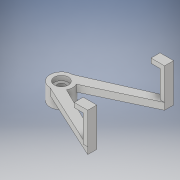
# Autodesk Inventor part: microphone_fix
Saved by Autodesk Inventor 2018 (Build 220112000, 112)
## iProperties
Created: 2018-02-07
Part Number: microphone_fix
Material: Generic
Document SubType Name: Modeling
Designer: Benedikt
Density: 1 g/cm^3
Appearance: Default
Author: Benedikt
## iProperties of the stored document microphone_fix_3DPrint.ipt
Created: 2018-02-14
Part Number: microphone_fix_3DPrint
Material: Generic
Document SubType Name: Modeling
Designer: Benedikt
Density: 1 g/cm^3
Appearance: Default
Author: Benedikt
Autodesk Inventor part; units mm, degrees
ref_plane "YZ Plane" through (0, 0, 0) normal (1, 0, 0) x (0, 1, 0)
ref_plane "XZ Plane" through (0, 0, 0) normal (0, 1, 0) x (-1, 0, 0)
ref_plane "XY Plane" through (0, 0, 0) normal (0, 0, 1) x (1, 0, 0)
sketch "Sketch1" plane through (0, 0, 0) normal (0, 0, 1) x (1, 0, 0)
  circle A0 centre (1.2, 90) radius 1.7 projected
  circle A1 centre (1.2, 90) radius 5
  point P0 (0, 0)
  dimension "d0" = 10
  constraints: 1 centre point, 1 coincident
  measures "d0" diameter of A1
extrude "Extrusion1" add sketch "Sketch1" along normal blind 4.5
sketch "Sketch2" plane through (1.2, 90, 4.5) normal (0, 0, 1) x (1, 0, 0)
  circle A0 centre (0, 0) radius 1.7 projected
  line L0 (31, 14.6742) -> (31, -15.3258) construction
  circle A1 centre (0, 0) radius 5 projected
  line L1 (31, 14.6742) -> (31, 18.6742)
  line L2 (31, 18.6742) -> (0, 5)
  line L3 (31, -15.3258) -> (31, -19.3258)
  line L4 (31, -19.3258) -> (0, -5)
  line L5 (31, 14.6742) -> (4.5193, 2.1392)
  line L6 (31, -15.3258) -> (4.4822, -2.2159)
  arc A2 (0, 5) -> (0, -5) centre (0, 0) ccw
  arc A3 (4.4822, -2.2159) -> (4.5193, 2.1392) centre (0, 0) ccw
  point P0 (-1.2, -90)
  dimension "d3" = 31
  dimension "d4" = 30
  dimension "d5" = 4
  dimension "d6" = 4
  constraints: 14 end point, 8 point on circle, 3 vertical, 2 centre point, 1 coincident
  measures "d3" distance from line of A0.centre L0
  measures "d4" distance of L0.end L0.start
  measures "d5" distance of L0.start L1.end
  measures "d6" distance of L0.end L3.end
extrude "Extrusion2" add sketch "Sketch2" along normal blind 3 contours A0 | A1 | A1 L2 L1 L5 | L6 L3 L4 A1
sketch "Sketch3" plane through (1.2, 90, 7.5) normal (0, 0, 1) x (1, 0, 0)
  circle A0 centre (0, 0) radius 1.7 projected
  point P0 (-1.2, -90)
  constraints: 1 coincident
hole "Hole1" at (1.2, 90, 7.5) direction (0, 0, -1) diameter 3.4 end through all counterbore diameter 6.2 counterbore depth 2
sketch "Sketch4" plane through (1.2, 90, 7.5) normal (0, 0, 1) x (1, 0, 0)
  line L0 (31, 18.6742) -> (0, 5) projected
  line L1 (31, 18.6742) -> (29, 18.6742)
  line L2 (29, 18.6742) -> (29, 14.6742)
  line L3 (29, 14.6742) -> (31, 14.6742)
  line L4 (31, 14.6742) -> (31, 18.6742)
  line L5 (31, -19.3258) -> (31, -15.3258) projected
  line L6 (31, -15.3258) -> (29, -15.3258)
  line L7 (29, -15.3258) -> (29, -19.3258)
  line L8 (29, -19.3258) -> (31, -19.3258)
  line L9 (31, -19.3258) -> (31, -15.3258)
  point P0 (-1.2, -90)
  dimension "d16" = 2
  dimension "d17" = 2
  constraints: 16 end point, 4 parallel, 2 horizontal, 2 perpendicular
  measures "d16" distance of L3.end L2.end
  measures "d17" distance of L8.end L7.end
extrude "Extrusion3" add sketch "Sketch4" along normal blind 14
sketch "Sketch5" plane through (30.2, 107.792, 7.5) normal (-1, 0, 0) x (0, 0, 1)
  line L0 (0, 0.8822) -> (14, 0.8822) projected
  line L1 (0, -3.1178) -> (14, -3.1178) projected
  line L2 (14, 0.8822) -> (12, 0.8822)
  line L3 (12, 0.8822) -> (12, -3.1178)
  line L4 (12, -3.1178) -> (14, -3.1178)
  line L5 (14, -3.1178) -> (14, 0.8822)
  line L6 (0, -33.1178) -> (14, -33.1178) projected
  line L7 (0, -37.1178) -> (14, -37.1178) projected
  line L8 (14, -33.1178) -> (12, -33.1178)
  line L9 (12, -33.1178) -> (12, -37.1178)
  line L10 (12, -37.1178) -> (14, -37.1178)
  line L11 (14, -37.1178) -> (14, -33.1178)
  point P0 (-7.5, -107.792)
  dimension "d20" = 2
  constraints: 16 end point, 4 parallel, 3 point on line, 2 horizontal, 2 perpendicular
  measures "d20" distance of L4.end L3.end
extrude "Extrusion4" add sketch "Sketch5" along normal blind 4
body "Solid1"
